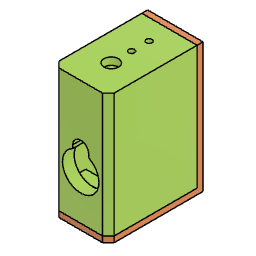
main (Autodesk Fusion 360 archive; units mm, degrees)
design "Leg"
Autodesk Fusion 360 part; units mm, degrees
sketch "スケッチ1" plane through (0, 0, 0) normal (0, 0, 1) x (1, 0, 0) in component "Component"
  line L0 (-100, 0) -> (100, 0)
  line L1 (0, 100) -> (0, -30)
  line L2 (-7.5, 0) -> (7.5, 0)
  line L3 (7.5, 0) -> (9.5, 2)
  line L4 (9.5, 2) -> (9.5, 30.5)
  line L5 (9.5, 30.5) -> (7.5, 30.5)
  line L6 (7.5, 30.5) -> (7.5, 4)
  line L7 (7.5, 4) -> (-7.5, 4)
  line L8 (-7.5, 4) -> (-7.5, 30.5)
  line L9 (-7.5, 30.5) -> (-9.5, 30.5)
  line L10 (-9.5, 30.5) -> (-9.5, 2)
  line L11 (-9.5, 2) -> (-7.5, 0)
  dimension "d1" = 15
  dimension "d2" = 45
  dimension "d3" = 2
  dimension "d4" = 4
  dimension "d5" = 26.5
  constraint horizontal L0
  constraint perpendicular L0 L1
  constraint coincident origin L0
  constraint coincident origin L1
  constraint coincident L0 L2.start
  constraint coincident L0 L2.end
  constraint perpendicular L0 L4
  constraint perpendicular L4 L5
  constraint perpendicular L5 L6
  constraint perpendicular L6 L7
  constraint perpendicular L7 L8
  constraint perpendicular L8 L9
  constraint perpendicular L0 L10
  constraint coincident L6.end L7.start
  constraint symmetric L1 L4 L10
  constraint symmetric L1 L6 L8
  constraint symmetric L1 L5 L9
  constraint symmetric L1 L3 L11
  constraint equal L2 L7
  measures "d1" distance of L6.end L7.end
  measures "d2" angle of L0 L3
  measures "d3" distance of L4 L6
  measures "d4" distance of origin L7
  measures "d5" distance of L7.end L8.end
extrude "押し出し1" add sketch "スケッチ1" along normal blind 2 makes body 1 in component "Component"
extrude "押し出し2" add sketch "スケッチ1" along normal blind 40 bodies 1 in component "Component"
sketch "スケッチ2" plane through (0, 4, 0) normal (0, 1, 0) x (-1, 0, 0) in component "Component"
  line L0 (7.5, 0) -> (7.5, 40)
  line L1 (7.5, 40) -> (-7.5, 40)
  line L2 (-7.5, 40) -> (-7.5, 0)
  line L3 (0, 40) -> (0, -34.75)
  line L4 (-6.25, 4.5) -> (6.25, 4.5)
  line L5 (6.25, 4.5) -> (6.25, 36.5)
  line L6 (6.25, 36.5) -> (-6.25, 36.5)
  line L7 (-6.25, 36.5) -> (-6.25, 4.5)
  line L8 (-6.25, 32) -> (6.25, 32)
  line L9 (6.25, 9) -> (-6.25, 9)
  line L10 (2.75, 22) -> (2.75, 20.8625)
  line L11 (-2.75, 22) -> (-2.75, 20.8625)
  arc A0 (-2.75, 20.8625) -> (2.75, 20.8625) centre (0, 15.25) ccw
  arc A1 (2.75, 22) -> (-2.75, 22) centre (0, 22) ccw
  circle A2 centre (0, 34.25) radius 1
  circle A3 centre (0, 6.75) radius 1
  line L12 (-7.5, 0) -> (7.5, 0)
  line L13 (-7.5, 0) -> (7.5, 0)
  dimension "d10" = 12.5
  dimension "d11" = 4.5
  dimension "d12" = 4.5
  dimension "d13" = 13
  dimension "d15" = 23
  dimension "d16" = 5.5
  dimension "d17" = 2
  dimension "d18" = 2.25
  dimension "d19" = 2.25
  dimension "d20" = 4.5
  constraint midpoint L1 L3.start
  constraint horizontal L4
  constraint vertical L5
  constraint horizontal L6
  constraint vertical L7
  constraint coincident L7 L8.start
  constraint coincident L5 L8.end
  constraint perpendicular L5 L8
  constraint coincident L5 L9.start
  constraint coincident L7 L9.end
  constraint perpendicular L5 L9
  constraint coincident L3 A0.centre
  constraint coincident L3 A1.centre
  constraint tangent L9 A0
  constraint tangent L5 A0
  constraint parallel L3 L10
  constraint parallel L3 L11
  constraint tangent L10 A1
  constraint tangent L11 A1
  constraint coincident L3 A2.centre
  constraint equal A2 A3
  constraint coincident L3 A3.centre
  measures "d10" distance of L4.start L4.end
  measures "d11" distance of L4 L9
  measures "d12" distance of L6 L8
  measures "d13" distance of L9 A1.centre
  measures "d15" distance of L8 L9
  measures "d16" diameter of A1
  measures "d17" diameter of A2
  measures "d18" distance of L6 A2.centre
  measures "d19" distance of L4 A3.centre
  measures "d20" distance of L4 L13
extrude "押し出し3" cut sketch "スケッチ2" against normal blind 23 contours L3 L11 A0 A1 | L3 L10 A0 A1 bodies 1 in component "Component"
extrude "押し出し4" add sketch "スケッチ2" along normal blind 4 contours L3 L4 L7 L9 A3 | L3 L4 L5 L9 A3 | L3 L5 L6 L8 A2 | L3 L6 L7 L8 A2 | L3 A3 | L3 A3 | L3 A2 | L3 A2 bodies 1 in component "Component"
extrude "押し出し5" cut sketch "スケッチ2" along normal blind 11 and the other way blind 2 contours L3 A3 | L3 A3 | L3 A2 | L3 A2 bodies 1 in component "Component"
sketch "スケッチ3" plane through (0, 0, 40) normal (0, 0, 1) x (-1, 0, 0) in component "Component"
  line L0 (9.5, -2) -> (7.5, 0)
  line L1 (7.5, 0) -> (-7.5, 0)
  line L2 (-7.5, 0) -> (-9.5, -2)
  line L3 (-9.5, -2) -> (-9.5, -30.5)
  line L4 (-9.5, -30.5) -> (-7.5, -30.5)
  line L5 (-7.5, -30.5) -> (-7.5, -4)
  line L6 (-7.5, -4) -> (7.5, -4)
  line L7 (7.5, -4) -> (7.5, -30.5)
  line L8 (7.5, -30.5) -> (9.5, -30.5)
  line L9 (9.5, -30.5) -> (9.5, -2)
  line L10 (-9.5, -30.5) -> (-9.5, -2)
  line L11 (-9.5, -2) -> (-7.5, 0)
  line L12 (-7.5, 0) -> (7.5, 0)
  line L13 (7.5, 0) -> (9.5, -2)
  line L14 (9.5, -2) -> (9.5, -30.5)
  line L15 (9.5, -30.5) -> (-9.5, -30.5)
  circle A0 centre (0, -10.5) radius 2.5
  circle A1 centre (0, -17.5) radius 1
  circle A2 centre (0, -23.5) radius 1
  line L16 (0, -35) -> (0, 5)
  dimension "d29" = 10.5
  dimension "d30" = 7
  dimension "d31" = 6
  dimension "d32" = 5
  dimension "d33" = 2
  constraint coincident L3.end L4.start
  constraint coincident L2.end L3.start
  constraint coincident L1.end L2.start
  constraint coincident L0.end L1.start
  constraint coincident L0.start L9.end
  constraint coincident L8.end L9.start
  constraint vertical L16
  constraint coincident origin L16
  constraint coincident A0.centre L16
  constraint coincident A1.centre L16
  constraint coincident A2.centre L16
  constraint equal A1 A2
  measures "d29" distance of L12 A0.centre
  measures "d30" distance of A0.centre A1.centre
  measures "d31" distance of A1.centre A2.centre
  measures "d32" diameter of A0
  measures "d33" diameter of A1
extrude "押し出し6" add sketch "スケッチ3" along normal blind 2.5 contours L0 L1 L6 L7 L8 L9 L12 L13 L14 L15 L16 | L1 L2 L3 L4 L5 L6 L10 L11 L12 L15 L16 | L6 L7 L15 A0 A1 A2 L16 | L5 L6 L15 A0 A1 A2 L16 bodies 1 in component "Component"
sketch "スケッチ4" plane through (0, 30.5, 0) normal (0, 1, 0) x (-1, 0, 0) in component "Component"
  line L0 (-9.5, 0) -> (-7.5, 0)
  line L1 (-7.5, 0) -> (-7.5, 40)
  line L2 (-7.5, 40) -> (7.5, 40)
  line L3 (7.5, 40) -> (7.5, 0)
  line L4 (7.5, 0) -> (9.5, 0)
  line L5 (9.5, 0) -> (9.5, 42.5)
  line L6 (9.5, 42.5) -> (-9.5, 42.5)
  line L7 (-9.5, 42.5) -> (-9.5, 0)
  circle A0 centre (-7, 40) radius 2.5
  line L8 (0, 55) -> (0, -6)
  circle A1 centre (7, 40) radius 2.5
  dimension "d37" = 5
  constraint tangent L6 A0
  constraint tangent L7 A0
  constraint vertical L8
  constraint coincident origin L8
  constraint symmetric A0 L8 A1
  measures "d37" diameter of A0
extrude "押し出し7" add sketch "スケッチ4" against normal up to surface (26.5 mm away) contours L1 L2 A0 | L2 L3 A1 picked at (-5.5091, 39.8774) picked at (5.5091, 39.8774) bodies 1 in component "Component"
sketch "スケッチ5" plane through (-9.5, 0, 0) normal (-1, 0, 0) x (0, -1, 0) in component "Component"
  line L0 (-30.5, 0) -> (-2, 0)
  line L1 (-2, 0) -> (-2, 42.5)
  line L2 (-2, 42.5) -> (-30.5, 42.5)
  line L3 (-30.5, 42.5) -> (-30.5, 0)
  circle A0 centre (-25.5, 5) radius 3
  line L4 (-26.25, 2.0953) -> (-26.25, 0)
  line L5 (-24.75, 2.0953) -> (-24.75, 0)
  line L6 (-25.5, 5) -> (-25.5, -4)
  line L7 (-24.75, 0) -> (-26.25, 0)
  dimension "d83" = 6
  dimension "d84" = 5
  dimension "d85" = 5
  dimension "d88" = 1.5
  constraint coincident A0 L4.start
  constraint coincident L0 L4.end
  constraint perpendicular L0 L4
  constraint coincident A0 L5.start
  constraint coincident L0 L5.end
  constraint perpendicular L0 L5
  constraint coincident A0.centre L6.start
  constraint vertical L6
  constraint symmetric L4 L5 L6
  measures "d83" diameter of A0
  measures "d84" distance of L0 A0.centre
  measures "d85" distance of L3 A0.centre
  measures "d88" distance of L4.end L5.end
extrude "押し出し9" cut sketch "スケッチ5" against normal blind 5 contours L0 A0 L4 L6 L7 | L0 A0 L5 L6 L7 | A0 bodies 1 in component "Component"
sketch "スケッチ1 (2)" plane through (0, 30.5, 0) normal (0, 1, 0) x (-1, 0, 0) in component "Component'"
  line L0 (-9.5, 0) -> (-7.5, 0)
  line L1 (-7.5, 0) -> (-7.5, 37.5505)
  line L2 (-4.5, 40) -> (4.5, 40)
  arc A0 (4.5, 40) -> (7.5, 37.5505) centre (7, 40) ccw
  line L3 (7.5, 37.5505) -> (7.5, 0)
  line L4 (7.5, 0) -> (9.5, 0)
  line L5 (9.5, 0) -> (9.5, 42.5)
  line L6 (9.5, 42.5) -> (-9.5, 42.5)
  line L7 (-9.5, 42.5) -> (-9.5, 0)
  line L8 (-9.5, 42.5) -> (9.5, 42.5)
  line L9 (9.5, 42.5) -> (9.5, -2)
  line L10 (9.5, -2) -> (-9.5, -2)
  line L11 (-9.5, -2) -> (-9.5, 42.5)
  arc A1 (-7.5, 37.5505) -> (-4.5, 40) centre (-7, 40) ccw
  dimension "d40" = 2
  constraint coincident L6.end L7.start
  constraint coincident L5.end L6.start
  constraint perpendicular L8 L9
  constraint perpendicular L9 L10
  constraint perpendicular L0 L11
  measures "d40" distance of L4.end L9.end
extrude "押し出し1'" add sketch "スケッチ1 (2)" along normal blind 2 separate body makes body 2 in component "Component'"
sketch "スケッチ2 (2)" plane through (0, 0, 0) normal (0, 0, -1) x (1, 0, 0) in component "Component'"
  line L0 (-7.5, 0) -> (-9.5, -2)
  line L1 (-9.5, -2) -> (-9.5, -24.75)
  line L2 (-7.5, -24.75) -> (-7.5, -4)
  line L3 (-7.5, -4) -> (7.5, -4)
  line L4 (7.5, -4) -> (7.5, -30.5)
  line L5 (7.5, -30.5) -> (9.5, -30.5)
  line L6 (9.5, -30.5) -> (9.5, -2)
  line L7 (9.5, -2) -> (7.5, 0)
  line L8 (7.5, 0) -> (-7.5, 0)
  line L9 (-9.5, -2) -> (-7.5, 0)
  line L10 (-7.5, 0) -> (7.5, 0)
  line L11 (7.5, 0) -> (9.5, -2)
  line L12 (9.5, -2) -> (9.5, -32.5)
  line L13 (9.5, -32.5) -> (-9.5, -32.5)
  line L14 (-9.5, -32.5) -> (-9.5, -2)
  line L15 (-9.5, -24.75) -> (-7.5, -24.75)
  point P0 (-9.5, -32.5)
  constraint coincident L0.end L1.start
  constraint coincident L0.start L8.end
  constraint coincident L7.end L8.start
  constraint coincident L6.end L7.start
  constraint perpendicular L8 L12
  constraint perpendicular L12 L13
  constraint coincident P0 L13.end
extrude "押し出し2'" add sketch "スケッチ2 (2)" along normal blind 2 bodies 2 in component "Component'"
sketch "スケッチ3 (2)" plane through (0, 32.5, 0) normal (0, 1, 0) x (-1, 0, 0) in component "Component'"
  line L0 (9.5, -2) -> (9.5, 42.5)
  line L1 (9.5, 42.5) -> (-9.5, 42.5)
  line L2 (-9.5, 42.5) -> (-9.5, -2)
  line L3 (-9.5, -2) -> (9.5, -2)
  line L4 (0, -10) -> (0, 50)
  circle A0 centre (0, 15.25) radius 1.65
  dimension "d71" = 17.25
  dimension "d72" = 3.3
  constraint perpendicular L1 L4
  constraint coincident origin L4
  constraint coincident L4 A0.centre
  measures "d71" distance of L3 A0.centre
  measures "d72" diameter of A0
extrude "押し出し3'" cut sketch "スケッチ3 (2)" against normal blind 5 contours L4 A0 | L4 A0 bodies 2 in component "Component'"
sketch "スケッチ1 (3)" plane through (0, 32.5, 0) normal (0, 1, 0) x (-1, 0, 0)
  line L0 (9.5, -2) -> (9.5, 42.5)
  line L1 (9.5, 42.5) -> (-9.5, 42.5)
  line L2 (-9.5, 42.5) -> (-9.5, -2)
  line L3 (-9.5, -2) -> (9.5, -2)
  circle A0 centre (-7, 40) radius 1
  circle A1 centre (7, 40) radius 1
  line L4 (0, 55) -> (0, -7)
  circle A2 centre (0, 15.25) radius 1.65
  dimension "d45" = 2.5
  dimension "d46" = 2.5
  dimension "d47" = 2
  constraint perpendicular L3 L4
  constraint coincident origin L4
  constraint symmetric A0 A1 L4
  measures "d45" distance of L1 A0.centre
  measures "d46" distance of L2 A0.centre
  measures "d47" diameter of A0
sketch "スケッチ2 (3)" plane through (0, 0, -2) normal (0, 0, -1) x (1, 0, 0)
  line L0 (-9.5, -2) -> (-9.5, -32.5)
  line L1 (-9.5, -32.5) -> (9.5, -32.5)
  line L2 (9.5, -32.5) -> (9.5, -2)
  line L3 (9.5, -2) -> (7.5, 0)
  line L4 (7.5, 0) -> (-7.5, 0)
  line L5 (-7.5, 0) -> (-9.5, -2)
  circle A0 centre (-6, -2) radius 1
  circle A1 centre (6, -2) radius 1
  line L6 (0, 14) -> (0, -36)
  dimension "d48" = 2
  dimension "d49" = 2
  dimension "d50" = 6
  constraint perpendicular L1 L6
  constraint coincident origin L6
  constraint symmetric A0 A1 L6
  measures "d48" distance of L4 A0.centre
  measures "d49" diameter of A0
  measures "d50" distance of A0.centre L6
hole "穴1" at (7, 32.5, 40) at (-7, 32.5, 40) direction (0, -1, 0) diameter 2 depth 8 tip angle 118 countersink diameter 4 countersink angle 90 bodies 1 in component "Component"
hole "穴1'" at (7, 32.5, 40) at (-7, 32.5, 40) direction (0, -1, 0) diameter 2 depth 8 tip angle 118 countersink diameter 4 countersink angle 90 bodies 2 in component "Component'"
hole "穴2" at (-6, 2, -2) at (6, 2, -2) direction (0, 0, 1) diameter 2 depth 8 tip angle 118 countersink diameter 4 countersink angle 90 bodies 1 in component "Component"
hole "穴2'" at (-6, 2, -2) at (6, 2, -2) direction (0, 0, 1) diameter 2 depth 8 tip angle 118 countersink diameter 4 countersink angle 90 bodies 2 in component "Component'"
component "Component" placed x (1, 0, 0) y (0, 1, 0) z (0, 0, 1) at (0, 0, 0)
component "Component'" placed x (1, 0, 0) y (0, 1, 0) z (0, 0, 1) at (0, 0, 0)

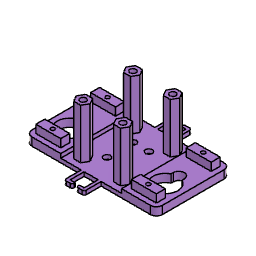
design "Body v2"
Autodesk Fusion 360 part; units mm, degrees
sketch "スケッチ1" plane through (0, 0, 0) normal (0, 0, 1) x (1, 0, 0) in component "Component"
  line L0 (-32.75, 0) -> (32.75, 0)
  line L1 (32.75, 0) -> (32.75, 37)
  line L2 (32.75, 37) -> (-32.75, 37)
  line L3 (-32.75, 37) -> (-32.75, 0)
  line L4 (0, 100) -> (0, -23.7582)
  line L5 (30.25, 34.5) -> (17.75, 34.5)
  line L6 (17.75, 34.5) -> (17.75, 2.5)
  line L7 (17.75, 2.5) -> (30.25, 2.5)
  line L8 (30.25, 2.5) -> (30.25, 34.5)
  line L9 (17.75, 30) -> (30.25, 30)
  line L10 (30.25, 7) -> (17.75, 7)
  line L11 (21.25, 20) -> (21.25, 18.8625)
  line L12 (26.75, 20) -> (26.75, 18.8625)
  circle A0 centre (24, 32.25) radius 1
  circle A1 centre (24, 4.75) radius 1
  line L13 (24, 34.5) -> (24, 2.5) construction
  line L14 (-17.75, 34.5) -> (-17.75, 2.5)
  line L15 (-17.75, 30) -> (-30.25, 30)
  line L16 (-30.25, 34.5) -> (-17.75, 34.5)
  line L17 (-21.25, 20) -> (-21.25, 18.8625)
  line L18 (-17.75, 2.5) -> (-30.25, 2.5)
  circle A2 centre (-24, 32.25) radius 1
  line L19 (-26.75, 20) -> (-26.75, 18.8625)
  circle A3 centre (-24, 4.75) radius 1
  line L20 (-30.25, 7) -> (-17.75, 7)
  line L21 (-30.25, 2.5) -> (-30.25, 34.5)
  line L22 (-24, 34.5) -> (-24, 2.5) construction
  arc A4 (21.25, 18.8625) -> (26.75, 18.8625) centre (24, 13.25) ccw
  arc A5 (26.75, 20) -> (21.25, 20) centre (24, 20) ccw
  arc A6 (-26.75, 18.8625) -> (-21.25, 18.8625) centre (-24, 13.25) ccw
  arc A7 (-21.25, 20) -> (-26.75, 20) centre (-24, 20) ccw
  line L23 (15.25, 37) -> (15.25, 0)
  line L24 (-15.25, 37) -> (-15.25, 0)
  line L25 (6.5359, 31) -> (8.2679, 28)
  line L26 (8.2679, 28) -> (11.7321, 28)
  line L27 (11.7321, 28) -> (13.4641, 31)
  line L28 (13.4641, 31) -> (11.7321, 34)
  line L29 (11.7321, 34) -> (8.2679, 34)
  line L30 (8.2679, 34) -> (6.5359, 31)
  line L31 (6.5359, 6) -> (8.2679, 3)
  line L32 (8.2679, 3) -> (11.7321, 3)
  line L33 (11.7321, 3) -> (13.4641, 6)
  line L34 (13.4641, 6) -> (11.7321, 9)
  line L35 (11.7321, 9) -> (8.2679, 9)
  line L36 (8.2679, 9) -> (6.5359, 6)
  line L37 (-13.4641, 31) -> (-11.7321, 34)
  line L38 (-11.7321, 28) -> (-13.4641, 31)
  line L39 (-8.2679, 28) -> (-11.7321, 28)
  line L40 (-6.5359, 31) -> (-8.2679, 28)
  line L41 (-11.7321, 34) -> (-8.2679, 34)
  line L42 (-8.2679, 34) -> (-6.5359, 31)
  line L43 (-6.5359, 6) -> (-8.2679, 3)
  line L44 (-8.2679, 3) -> (-11.7321, 3)
  line L45 (-11.7321, 3) -> (-13.4641, 6)
  line L46 (-8.2679, 9) -> (-6.5359, 6)
  line L47 (-13.4641, 6) -> (-11.7321, 9)
  line L48 (-11.7321, 9) -> (-8.2679, 9)
  line L49 (-3.5, 0) -> (-3.5, -7)
  line L50 (-3.5, -7) -> (-1, -7)
  line L51 (-1, -7) -> (-1, -8.5)
  line L52 (-1, -8.5) -> (-5, -8.5)
  line L53 (-5, -8.5) -> (-5, 0)
  line L54 (5, 0) -> (5, -8.5)
  line L55 (5, -8.5) -> (1, -8.5)
  line L56 (1, -8.5) -> (1, -7)
  line L57 (1, -7) -> (3.5, -7)
  line L58 (3.5, -7) -> (3.5, 0)
  circle A8 centre (4, 25) radius 1.7
  circle A9 centre (4, 12) radius 1.7
  circle A10 centre (-4, 25) radius 1.7
  circle A11 centre (-4, 12) radius 1.7
  line L59 (-44, 18.5) -> (109.5, 18.5) construction
  line L60 (3.5, 44) -> (3.5, 37)
  line L61 (5, 37) -> (5, 45.5)
  line L62 (1, 44) -> (3.5, 44)
  line L63 (-1, 44) -> (-1, 45.5)
  line L64 (-3.5, 44) -> (-1, 44)
  line L65 (-5, 45.5) -> (-5, 37)
  line L66 (-1, 45.5) -> (-5, 45.5)
  line L67 (1, 45.5) -> (1, 44)
  line L68 (5, 45.5) -> (1, 45.5)
  line L69 (-3.5, 37) -> (-3.5, 44)
  point P0 (10, 31)
  point P1 (10, 6)
  point P2 (-10, 31)
  point P3 (-10, 6)
  point P4 (0, 37)
  dimension "d1" = 12.5
  dimension "d2" = 4.5
  dimension "d3" = 4.5
  dimension "d4" = 2.5
  dimension "d5" = 13
  dimension "d6" = 5.5
  dimension "d7" = 2.5
  dimension "d9" = 23
  dimension "d10" = 2
  dimension "d11" = 2.25
  dimension "d12" = 2.25
  dimension "d13" = 48
  dimension "d14" = 2.5
  dimension "d15" = 2.5
  dimension "d27" = 10
  dimension "d28" = 10
  dimension "d29" = 25
  dimension "d30" = 6
  dimension "d33" = 6
  dimension "d34" = 6
  dimension "d38" = 7
  dimension "d39" = 1.5
  dimension "d40" = 1.5
  dimension "d41" = 7
  dimension "d42" = 2
  dimension "d43" = 3.4
  dimension "d44" = 8
  dimension "d45" = 8
  dimension "d46" = 12
  dimension "d47" = 12
  constraint horizontal L0
  constraint vertical L1
  constraint horizontal L2
  constraint vertical L3
  constraint perpendicular L0 L4
  constraint coincident origin L4
  constraint coincident origin L0
  constraint horizontal L5
  constraint vertical L6
  constraint horizontal L7
  constraint vertical L8
  constraint coincident L6 L9.start
  constraint coincident L8 L9.end
  constraint perpendicular L8 L9
  constraint coincident L8 L10.start
  constraint coincident L6 L10.end
  constraint perpendicular L6 L10
  constraint tangent L10 A4
  constraint tangent L8 A4
  constraint tangent L6 A4
  constraint tangent L11 A5
  constraint vertical L11
  constraint tangent L12 A5
  constraint equal L11 L12
  constraint vertical L12
  constraint perpendicular L5 L13
  constraint midpoint L5 L13.start
  constraint midpoint L7 L13.end
  constraint coincident A1.centre L13
  constraint coincident A0.centre L13
  constraint symmetric L4 L5.start L16.start
  constraint symmetric L4 L5.end L14.start
  constraint symmetric L4 L6.end L14.end
  constraint symmetric L4 L7.end L18.end
  constraint symmetric L4 L9.start L15.start
  constraint symmetric L4 L9.end L15.end
  constraint symmetric L4 L10.start L20.start
  constraint symmetric L4 L10.end L20.end
  constraint symmetric L4 A4 A6
  constraint symmetric L4 A5 A7
  constraint symmetric L4 L11.start L17.start
  constraint symmetric L4 L11.end L17.end
  constraint symmetric L4 L12.start L19.start
  constraint symmetric L4 L12.end L19.end
  constraint symmetric L4 A0 A2
  constraint symmetric L4 A1 A3
  constraint symmetric L4 L13.start L22.start
  constraint symmetric L4 L13.end L22.end
  constraint equal A0 A1
  constraint coincident L2 L23.start
  constraint coincident L0 L23.end
  constraint perpendicular L0 L23
  constraint coincident L2 L24.start
  constraint coincident L0 L24.end
  constraint perpendicular L0 L24
  constraint horizontal L32
  constraint horizontal L26
  constraint symmetric L4 L25.start L40.start
  constraint symmetric L4 L25.end L39.start
  constraint symmetric L4 L26.end L38.start
  constraint symmetric L4 L27.end L37.start
  constraint symmetric L4 L28.end L37.end
  constraint symmetric L4 L29.end L41.end
  constraint symmetric L4 P0 P2
  constraint symmetric L4 L31.start L43.start
  constraint symmetric L4 L31.end L43.end
  constraint symmetric L4 L32.end L44.end
  constraint symmetric L4 L33.end L45.end
  constraint symmetric L4 L34.end L47.end
  constraint symmetric L4 L35.end L46.start
  constraint symmetric L4 P1 P3
  constraint perpendicular L2 L49
  constraint perpendicular L4 L50
  constraint perpendicular L2 L51
  constraint perpendicular L4 L52
  constraint perpendicular L2 L53
  constraint perpendicular L0 L54
  constraint perpendicular L54 L55
  constraint perpendicular L55 L56
  constraint perpendicular L56 L57
  constraint coincident L0 L58.end
  constraint perpendicular L0 L58
  constraint symmetric L4 L53 L54
  constraint collinear L50 L57
  constraint collinear L52 L55
  constraint coincident L0 L49.start
  constraint symmetric L4 L51 L56
  constraint equal A8 A9
  constraint symmetric L4 A8 A10
  constraint symmetric L4 A9 A11
  constraint horizontal L59
  constraint midpoint L1 L59
  constraint symmetric origin L59 P4
  constraint symmetric L49.start L59 L69.start
  constraint symmetric L49.end L59 L64.start
  constraint symmetric L50.end L59 L63.start
  constraint symmetric L51.end L59 L63.end
  constraint symmetric L52.end L59 L65.start
  constraint symmetric L53.end L59 L65.end
  constraint symmetric L54.start L59 L61.start
  constraint symmetric L54.end L59 L61.end
  constraint symmetric L55.end L59 L67.start
  constraint symmetric L56.end L59 L62.start
  constraint symmetric L57.end L59 L60.start
  constraint symmetric L58.end L59 L60.end
  measures "d1" distance of L6.end L7.end
  measures "d2" distance of L7 L10
  measures "d3" distance of L5 L9
  measures "d4" distance of L0 L7
  measures "d5" distance of L10 A5.centre
  measures "d6" diameter of A5
  measures "d7" distance of L1 L8
  measures "d9" distance of L9.start L10.end
  measures "d10" diameter of A0
  measures "d11" distance of L5 A0.centre
  measures "d12" distance of L7 A1.centre
  measures "d13" distance of A4.centre A6.centre
  measures "d14" distance of L2 L5
  measures "d15" distance of L5.end L23
  measures "d27" distance of L4 P0
  measures "d28" distance of L4 P1
  measures "d29" distance of P0 P1
  measures "d30" distance of L2 P0
  measures "d33" distance of L26 L29
  measures "d34" distance of L32 L35
  measures "d38" distance of L49 L58
  measures "d39" distance of L54 L58
  measures "d40" distance of L50.end L51.end
  measures "d41" distance of L49.start L49.end
  measures "d42" distance of L51 L56
  measures "d43" diameter of A9
  measures "d44" distance of A8.centre A10.centre
  measures "d45" distance of A9.centre A11.centre
  measures "d46" distance of L2 A10.centre
  measures "d47" distance of L0 A11.centre
extrude "押し出し1" add sketch "スケッチ1" along normal blind 4 contours L0 L2 L3 L24 | L0 L1 L2 L23 | L6 L8 L9 L11 L12 A4 A5 | L8 L10 A4 | L6 L10 A4 | L14 L15 L17 L19 L21 A6 A7 | L14 L20 A6 | L20 L21 A6 makes body 1 at (-24.0685, 27.5808, 0) makes body 2 at (24.0685, 27.5808, 4) in component "Component"
extrude "押し出し2" add sketch "スケッチ1" along normal blind 8 contours L5 L6 L8 L9 | L6 L7 L8 L10 | L14 L15 L16 L21 | L14 L18 L20 L21 bodies 1 2 in component "Component"
extrude "押し出し3" add sketch "スケッチ1" along normal blind 2 contours L0 L2 L4 L24 | L0 L2 L4 L23 | L25 L26 L27 L28 L29 L30 | L31 L32 L33 L34 L35 L36 | L37 L38 L39 L40 L41 L42 | L43 L44 L45 L46 L47 L48 | A8 | A9 | A10 | A11 bodies 1 2 in component "Component"
fillet "フィレット2" radius 3 4 edges at (-32.75, 0, 2) (32.75, 0, 2) (32.75, 37, 2) (-32.75, 37, 2) on bodies 1 in component "Component"
extrude "押し出し4" add sketch "スケッチ1" along normal blind 27 contours L25 L26 L27 L28 L29 L30 | L31 L32 L33 L34 L35 L36 | L37 L38 L39 L40 L41 L42 | L43 L44 L45 L46 L47 L48 bodies 1 in component "Component"
sketch "スケッチ2" plane through (0, 0, 27) normal (0, 0, 1) x (-1, 0, 0) in component "Component"
  line L0 (-8.2679, -34) -> (-6.5359, -31)
  line L1 (-6.5359, -31) -> (-8.2679, -28)
  line L2 (-8.2679, -28) -> (-11.7321, -28)
  line L3 (-11.7321, -28) -> (-13.4641, -31)
  line L4 (-13.4641, -31) -> (-11.7321, -34)
  line L5 (-11.7321, -34) -> (-8.2679, -34)
  circle A0 centre (-10, -31) radius 1.5
  line L6 (-8.2679, -34) -> (-11.7321, -28) construction
  line L7 (-11.7321, -34) -> (-8.2679, -28) construction
  line L8 (-8.2679, -9) -> (-11.7321, -3) construction
  line L9 (-11.7321, -9) -> (-8.2679, -3) construction
  circle A1 centre (-10, -6) radius 1.5
  line L10 (0, -52) -> (0, 9)
  circle A2 centre (10, -6) radius 1.5
  circle A3 centre (10, -31) radius 1.5
  point P0 (-8.2679, -9)
  point P1 (-11.7321, -9)
  point P2 (-11.7321, -3)
  point P3 (-8.2679, -3)
  dimension "d35" = 3
  constraint coincident L0.start L5.end
  constraint coincident L2.end L3.start
  constraint coincident L4.end L5.start
  constraint coincident L1.end L2.start
  constraint coincident A0.centre L6
  constraint coincident A0.centre L7
  constraint coincident P0 L8.start
  constraint coincident P1 L9.start
  constraint coincident P2 L8.end
  constraint coincident P3 L9.end
  constraint midpoint L8 A1.centre
  constraint equal A0 A1
  constraint vertical L10
  constraint coincident origin L10
  constraint symmetric A0 L10 A3
  constraint symmetric A1 L10 A2
  measures "d35" diameter of A0
extrude "押し出し5" cut sketch "スケッチ2" against normal blind 15 contours A0 | A1 | A2 | A3 bodies 1 in component "Component"
extrude "押し出し6" add sketch "スケッチ1" along normal up to surface (2 mm away) contours L0 L49 L50 L51 L52 L53 | L2 L63 L64 L65 L66 L69 | L0 L54 L55 L56 L57 L58 | L2 L60 L61 L62 L67 L68 bodies 1 in component "Component"
extrude "押し出し7" cut sketch "スケッチ1" along normal blind 11 contours A8 | A9 | A10 | A11 bodies 1 in component "Component"
fillet "フィレット3" radius 1 8 edges at (-5, -8.5, 1) (-1, -8.5, 1) (1, -8.5, 1) (5, -8.5, 1) (-5, 45.5, 1) (-1, 45.5, 1) (1, 45.5, 1) (5, 45.5, 1) on bodies 1 in component "Component"
component "Component" placed x (1, 0, 0) y (0, 1, 0) z (0, 0, 1) at (0, 0, 0)

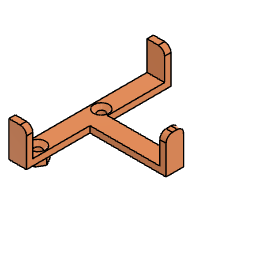
design "Micon Cace ver1"
Autodesk Fusion 360 part; units mm, degrees
sketch "スケッチ1" plane through (0, 0, 0) normal (0, 0, 1) x (1, 0, 0) in component "Component"
  line L0 (-3.4641, 12.5) -> (-1.7321, 9.5)
  line L1 (-1.7321, 9.5) -> (1.7321, 9.5)
  line L2 (1.7321, 9.5) -> (3.4641, 12.5)
  line L3 (3.4641, 12.5) -> (1.7321, 15.5)
  line L4 (1.7321, 15.5) -> (-1.7321, 15.5)
  line L5 (-1.7321, 15.5) -> (-3.4641, 12.5)
  line L6 (0, 150) -> (0, -150) construction
  line L7 (-100, 0) -> (234.7346, 0) construction
  line L8 (-3.4641, -12.5) -> (-1.7321, -9.5)
  line L9 (-1.7321, -9.5) -> (1.7321, -9.5)
  line L10 (3.4641, -12.5) -> (1.7321, -15.5)
  line L11 (-1.7321, -15.5) -> (-3.4641, -12.5)
  line L12 (1.7321, -9.5) -> (3.4641, -12.5)
  line L13 (1.7321, -15.5) -> (-1.7321, -15.5)
  line L14 (-31, 8) -> (50, 8)
  line L15 (-3.4641, 12.5) -> (-3.4641, 34)
  line L16 (-3.4641, 34) -> (3.4641, 34)
  line L17 (3.4641, 34) -> (3.4641, -18)
  line L18 (3.4641, -18) -> (-3.4641, -18)
  line L19 (-3.4641, -18) -> (-3.4641, 12.5)
  line L20 (-3.4641, 34) -> (-3.4641, 36.5)
  line L21 (-3.4641, 36.5) -> (3.4641, 36.5)
  line L22 (3.4641, 36.5) -> (3.4641, 34)
  line L23 (-3.4641, -18) -> (-3.4641, -20.5)
  line L24 (-3.4641, -20.5) -> (3.4641, -20.5)
  line L25 (3.4641, -20.5) -> (3.4641, -18)
  line L26 (3.4641, 11.4641) -> (31, 11.4641)
  line L27 (31, 11.4641) -> (31, 4.5359)
  line L28 (31, 4.5359) -> (3.4641, 4.5359)
  line L29 (31, 11.4641) -> (33.5, 11.4641)
  line L30 (33.5, 11.4641) -> (33.5, 4.5359)
  line L31 (33.5, 4.5359) -> (31, 4.5359)
  point P0 (0, 12.5)
  point P1 (0, -12.5)
  dimension "d1" = 6
  dimension "d2" = 25
  dimension "d3" = 8
  dimension "d4" = 52
  dimension "d5" = 2.5
  dimension "d6" = 2.5
  dimension "d7" = 31
  constraint vertical L6
  constraint coincident origin L6
  constraint coincident P0 L6
  constraint perpendicular L6 L7
  constraint coincident origin L7
  constraint symmetric L0.start L7 L8.start
  constraint symmetric L0.end L7 L8.end
  constraint symmetric L1.end L7 L9.end
  constraint symmetric L2.end L7 L10.start
  constraint symmetric L3.end L7 L10.end
  constraint symmetric L4.end L7 L11.start
  constraint symmetric P0 L7 P1
  constraint horizontal L14
  constraint vertical L15
  constraint perpendicular L15 L16
  constraint perpendicular L16 L17
  constraint perpendicular L17 L18
  constraint perpendicular L18 L19
  constraint coincident L2.end L17
  constraint symmetric L14 L16 L18
  constraint perpendicular L16 L20
  constraint perpendicular L20 L21
  constraint perpendicular L18 L23
  constraint perpendicular L23 L24
  constraint vertical L22
  constraint vertical L25
  constraint coincident L17 L26.start
  constraint perpendicular L17 L26
  constraint perpendicular L26 L27
  constraint coincident L17 L28.end
  constraint perpendicular L17 L28
  constraint symmetric L14 L26 L28
  constraint equal L21 L27
  constraint perpendicular L27 L29
  constraint perpendicular L26 L30
  constraint horizontal L31
  constraint equal L22 L29
  measures "d1" distance of L0 L3
  measures "d2" distance of P0 P1
  measures "d3" distance of L7 L14.end
  measures "d4" distance of L16 L18
  measures "d5" distance of L16.end L21.end
  measures "d6" distance of L17.end L24.end
  measures "d7" distance of L6 L27
extrude "押し出し1" add sketch "スケッチ1" against normal blind 2.5 contours L0 L1 L2 L3 L4 L5 | L8 L9 L10 L11 L12 L13 makes body 1 at (-0.5774, 11.5, 0) makes body 2 at (-0.5774, -11.5, 0) in component "Component"
extrude "押し出し2" add sketch "スケッチ1" along normal blind 2.5 contours L0 L1 L2 L3 L4 L5 | L3 L4 L5 L15 L16 L17 | L0 L1 L2 L14 L17 L19 | L8 L9 L12 L14 L17 L19 | L14 L17 L26 L27 | L14 L17 L27 L28 | L8 L9 L10 L11 L12 L13 | L10 L11 L13 L17 L18 L19 bodies 1 2 in component "Component"
extrude "押し出し3" add sketch "スケッチ1" along normal blind 14 contours L16 L20 L21 L22 | L14 L27 L29 L30 | L14 L27 L30 L31 | L18 L23 L24 L25 bodies 1 in component "Component"
sketch "スケッチ2" plane through (0, 0, 2.5) normal (0, 0, 1) x (-1, 0, 0) in component "Component"
  line L0 (-31, -4.5359) -> (-31, -11.4641)
  line L1 (-31, -11.4641) -> (-3.4641, -11.4641)
  line L2 (-3.4641, -11.4641) -> (-3.4641, -34)
  line L3 (-3.4641, -34) -> (3.4641, -34)
  line L4 (3.4641, -34) -> (3.4641, 18)
  line L5 (3.4641, 18) -> (-3.4641, 18)
  line L6 (-3.4641, 18) -> (-3.4641, -4.5359)
  line L7 (-3.4641, -4.5359) -> (-31, -4.5359)
  circle A0 centre (0, -12.5) radius 1.5
  circle A1 centre (0, 12.5) radius 1.5
  point P0 (0, -12.5)
  point P1 (0, 12.5)
  dimension "d14" = 3
  constraint equal A0 A1
  constraint coincident P0 A0.centre
  constraint coincident P1 A1.centre
  measures "d14" diameter of A0
hole "穴1" at (0, 12.5, 2.5) at (0, -12.5, 2.5) direction (0, 0, -1) diameter 3 depth 10 tip angle 118 countersink diameter 6 countersink angle 90 bodies 1 in component "Component"
fillet "フィレット1" radius 2.5 4 edges at (3.4641, 35.25, 14) (3.4641, -19.25, 14) (32.25, 4.5359, 14) (32.25, 11.4641, 14) on bodies 1 in component "Component"
component "Component" placed x (1, 0, 0) y (0, 1, 0) z (0, 0, 1) at (0, 0, 0)

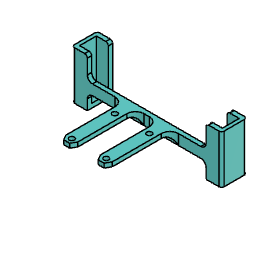
design "Micon Cace sub"
Autodesk Fusion 360 part; units mm, degrees
ref_plane "作業平面1" through (41.5, 0, 0) normal (1, 0, 0) x (0, 1, 0) in component "Component"
sketch "スケッチ1" plane through (41.5, 0, 0) normal (1, 0, 0) x (0, 1, 0) in component "Component"
  line L0 (0, 0) -> (0, 28)
  line L1 (0, 28) -> (2.5, 28)
  line L2 (2.5, 28) -> (2.5, 2.5)
  line L3 (2.5, 2.5) -> (12.25, 2.5)
  line L4 (12.25, 2.5) -> (12.25, 28)
  line L5 (12.25, 28) -> (14.75, 28)
  line L6 (14.75, 28) -> (14.75, 0)
  line L7 (14.75, 0) -> (0, 0)
  dimension "d2" = 28
  dimension "d3" = 2.5
  dimension "d4" = 9.75
  dimension "d5" = 2.5
  constraint coincident L0.start L7.end
  constraint vertical L0
  constraint perpendicular L0 L1
  constraint perpendicular L1 L2
  constraint perpendicular L2 L3
  constraint perpendicular L3 L4
  constraint perpendicular L4 L5
  constraint perpendicular L5 L6
  constraint perpendicular L0 L7
  constraint equal L2 L4
  constraint equal L1 L5
  measures "d2" distance of L0.start L0.end
  measures "d3" distance of L0.end L1.end
  measures "d4" distance of L2.end L3.end
  measures "d5" distance of L3 L7
extrude "押し出し1" add sketch "スケッチ1" against normal blind 7 makes body 1 in component "Component"
sketch "スケッチ4" plane through (41.5, 0, 0) normal (1, 0, 0) x (0, 1, 0) in component "Component"
  line L0 (14.75, 0) -> (14.75, 28)
  line L1 (14.75, 28) -> (12.25, 28)
  line L2 (12.25, 28) -> (12.25, 2.5)
  line L3 (12.25, 2.5) -> (2.5, 2.5)
  line L4 (2.5, 2.5) -> (2.5, 28)
  line L5 (2.5, 28) -> (0, 28)
  line L6 (0, 28) -> (0, 0)
  line L7 (0, 0) -> (14.75, 0)
  line L8 (0, 28) -> (14.75, 28)
  line L9 (14.75, 28) -> (14.75, 0)
  line L10 (14.75, 0) -> (0, 0)
  line L11 (0, 0) -> (0, 28)
  constraint horizontal L8
  constraint vertical L9
  constraint horizontal L10
  constraint vertical L11
  constraint coincident L0.start L7.end
  constraint coincident L5.end L6.start
extrude "押し出し4" add sketch "スケッチ4" along normal blind 2 bodies 1 in component "Component"
mirror "ミラー1" about plane through (0, 0, 0) normal (1, 0, 0) of bodies 1 makes body 2 in component "Component"
sketch "スケッチ2" plane through (0, 0, 0) normal (0, -1, 0) x (1, 0, 0) in component "Component"
  line L0 (34.5, 0) -> (43.5, 0)
  line L1 (34.5, 28) -> (34.5, 0)
  line L2 (43.5, 28) -> (34.5, 28)
  line L3 (34.5, 15) -> (-34.5, 15)
  line L4 (-34.5, 15) -> (-34.5, 9)
  line L5 (-34.5, 9) -> (34.5, 9)
  line L6 (-34.5, 28) -> (-34.5, 0)
  line L7 (34.5, 15) -> (41.5, 15)
  line L8 (41.5, 9) -> (34.5, 9)
  line L9 (41.5, 15) -> (41.5, 9)
  line L10 (-34.5, 15) -> (-41.5461, 15)
  line L11 (-41.5461, 15) -> (-41.5461, 9)
  line L12 (-41.5461, 9) -> (-34.5, 9)
  line L13 (43.5, 0) -> (43.5, 28)
  dimension "d24" = 6
  constraint horizontal L3
  constraint vertical L4
  constraint horizontal L5
  constraint coincident L1 L3.start
  constraint coincident L4.end L6
  constraint perpendicular L6 L10
  constraint perpendicular L10 L11
  measures "d24" distance of L7.end L8.start
extrude "押し出し2" add sketch "スケッチ2" against normal up to surface (2.5 mm away) contours L1 L3 L4 L5 L6 bodies 1 2 in component "Component"
sketch "スケッチ3" plane through (0, 0, 15) normal (0, 0, 1) x (-1, 0, 0) in component "Component"
  line L0 (-34.5, -2.5) -> (34.5, -2.5)
  line L1 (34.5, -2.5) -> (34.5, 0)
  line L2 (34.5, 0) -> (-34.5, 0)
  line L3 (-34.5, 0) -> (-34.5, -2.5)
  line L4 (0, -33) -> (0, 45)
  line L5 (-13.4641, 0) -> (-6.5359, 0)
  line L6 (-6.5359, 0) -> (-6.5359, 33.5)
  line L7 (-10, 67.917) -> (-13.4641, 67.917)
  line L8 (-13.4641, 33.5) -> (-13.4641, 0)
  circle A0 centre (-10, 8.5) radius 1.5
  circle A1 centre (-10, 33.5) radius 1.5
  line L9 (-8.2679, 30.5) -> (-6.5359, 33.5)
  line L10 (-6.5359, 33.5) -> (-8.2679, 36.5)
  line L11 (-8.2679, 36.5) -> (-11.7321, 36.5)
  line L12 (-11.7321, 36.5) -> (-13.4641, 33.5)
  line L13 (-13.4641, 33.5) -> (-11.7321, 30.5)
  line L14 (-11.7321, 30.5) -> (-8.2679, 30.5)
  line L15 (-10, 0) -> (-10, 36.5)
  line L16 (11.7321, 30.5) -> (8.2679, 30.5)
  line L17 (8.2679, 36.5) -> (11.7321, 36.5)
  circle A2 centre (10, 33.5) radius 1.5
  line L18 (8.2679, 30.5) -> (6.5359, 33.5)
  circle A3 centre (10, 8.5) radius 1.5
  line L19 (11.7321, 36.5) -> (13.4641, 33.5)
  line L20 (10, 0) -> (10, 36.5)
  line L21 (13.4641, 33.5) -> (11.7321, 30.5)
  line L22 (13.4641, 0) -> (6.5359, 0)
  line L23 (6.5359, 33.5) -> (8.2679, 36.5)
  line L24 (13.4641, 33.5) -> (13.4641, 0)
  line L25 (6.5359, 0) -> (6.5359, 33.5)
  point P0 (-10, 33.5)
  point P1 (10, 33.5)
  dimension "d15" = 8.5
  dimension "d16" = 25
  dimension "d18" = 3
  dimension "d19" = 6
  dimension "d21" = 10
  constraint vertical L4
  constraint coincident origin L4
  constraint horizontal L5
  constraint vertical L6
  constraint horizontal L7
  constraint vertical L8
  constraint coincident L2 L5.start
  constraint equal A0 A1
  constraint coincident P0 A1.centre
  constraint midpoint L5 L15.start
  constraint midpoint L11 L15.end
  constraint vertical L15
  constraint coincident A0.centre L15
  constraint symmetric L4 L5.start L22.start
  constraint symmetric L4 L5.end L22.end
  constraint symmetric L4 A0 A3
  constraint symmetric L4 A1 A2
  constraint symmetric L4 L9.start L16.end
  constraint symmetric L4 L6.end L18.end
  constraint symmetric L4 L10.end L17.start
  constraint symmetric L4 L11.end L17.end
  constraint symmetric L4 L8.start L19.end
  constraint symmetric L4 L13.end L16.start
  constraint symmetric L4 P0 P1
  constraint symmetric L4 L15.start L20.start
  constraint symmetric L4 L15.end L20.end
  measures "d15" distance of L5 A0.centre
  measures "d16" distance of A0.centre P0
  measures "d18" diameter of A0
  measures "d19" distance of L11 L14
  measures "d21" distance of origin L15.start
extrude "押し出し3" add sketch "スケッチ3" against normal blind 2.5 contours L2 L5 L8 A0 L13 L14 L15 | L2 L16 L18 A3 L20 L22 L25 | L2 L5 L6 A0 L9 L14 L15 | A1 L11 L12 L13 L14 L15 | L2 L16 A3 L20 L21 L22 L24 | L16 L17 A2 L18 L20 L23 | A1 L9 L10 L11 L14 L15 | L16 L17 A2 L19 L20 L21 bodies 1 in component "Component"
fillet "フィレット1" radius 3.5 2 edges at (-10, 0, 12.5) (10, 0, 12.5) on bodies 1 in component "Component"
fillet "フィレット2" radius 5 4 edges at (-6.5359, 0, 12) (13.4641, 0, 12) (6.5359, 0, 12) (-13.4641, 0, 12) on bodies 1 in component "Component"
fillet "フィレット3" radius 3 4 edges at (-34.5, 1.25, 15) (34.5, 1.25, 15) (-34.5, 1.25, 9) (34.5, 1.25, 9) on bodies 1 in component "Component"
fillet "フィレット4" radius 1.5 4 edges at (-34.5, 1.25, 28) (-34.5, 13.5, 28) (34.5, 1.25, 28) (34.5, 13.5, 28) on bodies 1 in component "Component"
fillet "フィレット5" radius 1.5 4 edges at (43.5, 14.75, 14) (43.5, 0, 14) (-43.5, 14.75, 14) (-43.5, 0, 14) on bodies 1 in component "Component"
component "Component" placed x (1, 0, 0) y (0, 1, 0) z (0, 0, 1) at (0, 0, 0)
